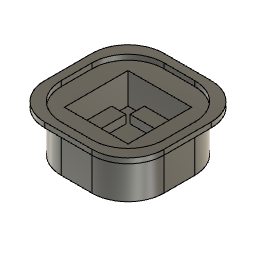
buttonCap (Autodesk Fusion 360 design; units mm, degrees)
Autodesk Fusion 360 part; units mm, degrees
sketch "Esquisse1" plane through (0, 0, 0) normal (0, 0, 1) x (1, 0, 0)
  line L0 (3.5, 0) -> (6.5, 0)
  line L1 (10, -3.5) -> (10, -6.5)
  line L2 (6.5, -10) -> (3.5, -10)
  line L3 (0, -6.5) -> (0, -3.5)
  arc A0 (3.5, 0) -> (0, -3.5) centre (3.5, -3.5) ccw
  arc A1 (10, -3.5) -> (6.5, 0) centre (6.5, -3.5) ccw
  arc A2 (6.5, -10) -> (10, -6.5) centre (6.5, -6.5) ccw
  arc A3 (0, -6.5) -> (3.5, -10) centre (3.5, -6.5) ccw
  point P0 (10, 0)
  point P1 (0, -10)
  dimension "d2" = 10
  dimension "d3" = 10
  dimension "d4" = 3.5
  dimension "d6" = 3.5
  dimension "d7" = 3.5
  dimension "d8" = 3.5
  constraint horizontal L0
  constraint vertical L1
  constraint horizontal L2
  constraint vertical L3
  constraint coincident origin L0
  constraint coincident origin L3
  constraint tangent L0 A0
  constraint tangent L3 A0
  constraint coincident P0 L0
  constraint coincident P0 L1
  constraint tangent L0 A1
  constraint tangent L1 A1
  constraint tangent L1 A2
  constraint tangent L2 A2
  constraint coincident P1 L2
  constraint coincident P1 L3
  constraint tangent L2 A3
  constraint tangent L3 A3
  measures "d2" distance of origin P0
  measures "d3" distance of origin P1
  measures "d4" radius of A0
  measures "d6" radius of A1
  measures "d7" radius of A2
  measures "d8" radius of A3
extrude "Extrusion1" add sketch "Esquisse1" along normal blind 4
ref_plane "Plan de construction1" through (0, 0, 4) normal (0, 0, 1) x (1, 0, 0)
sketch "button" plane through (0, 0, 4) normal (0, 0, 1) x (1, 0, 0)
  line L0 (0, 0) -> (1.9, 0) construction
  line L1 (0, 0) -> (0, -1.9) construction
  line L2 (1.9, 0) -> (1.9, -10) construction
  line L3 (0, -1.9) -> (10, -1.9) construction
  line L4 (1.9, -1.9) -> (8.1, -1.9)
  line L5 (8.1, -1.9) -> (8.1, -8.1)
  line L6 (8.1, -8.1) -> (1.9, -8.1)
  line L7 (1.9, -8.1) -> (1.9, -1.9)
  point P0 (1.9, -1.9)
  dimension "d14" = 1.9
  dimension "d15" = 1.9
  dimension "d16" = 10
  dimension "d17" = 10
  dimension "d18" = 6.2
  dimension "d19" = 6.2
  constraint coincident L0.start L1.start
  constraint horizontal L0
  constraint perpendicular L0 L1
  constraint perpendicular L0 L2
  constraint perpendicular L1 L3
  constraint coincident L2 P0
  constraint coincident L3 P0
  constraint horizontal L4
  constraint vertical L5
  constraint horizontal L6
  constraint vertical L7
  constraint coincident P0 L4.start
  measures "d14" distance of L0.start L0.end
  measures "d15" distance of L0.start L1.end
  measures "d16" distance of L0.end L2.end
  measures "d17" distance of L1.end L3.end
  measures "d18" distance of P0 L4.end
  measures "d19" distance of P0 L6.end
extrude "Extrude2" cut sketch "button" against normal blind 3
ref_plane "WorkPlane2" through (0, 0, 1) normal (0, 0, 1) x (1, 0, 0)
sketch "buttonHolder" plane through (0, 0, 1) normal (0, 0, 1) x (1, 0, 0)
  line L0 (0, 0) -> (3.5, 0) construction
  line L1 (0, 0) -> (0, -1.9) construction
  line L2 (3.5, 0) -> (3.5, -10) construction
  line L3 (0, -1.9) -> (10, -1.9) construction
  line L4 (3.5, -1.9) -> (6.5, -1.9)
  line L5 (6.5, -1.9) -> (6.5, -3.3)
  line L6 (6.5, -3.3) -> (3.5, -3.3)
  line L7 (3.5, -3.3) -> (3.5, -1.9)
  line L8 (0, 0) -> (0, -8.1) construction
  line L9 (0, -8.1) -> (10, -8.1) construction
  line L10 (3.5, -8.1) -> (6.5, -8.1)
  line L11 (6.5, -8.1) -> (6.5, -6.7)
  line L12 (6.5, -6.7) -> (3.5, -6.7)
  line L13 (3.5, -6.7) -> (3.5, -8.1)
  line L14 (0, 0) -> (1.9, 0) construction
  line L15 (1.9, 0) -> (1.9, -3.5) construction
  line L16 (1.9, -3.5) -> (3.3, -3.5)
  line L17 (3.3, -3.5) -> (3.3, -6.5)
  line L18 (3.3, -6.5) -> (1.9, -6.5)
  line L19 (1.9, -6.5) -> (1.9, -3.5)
  line L20 (0, 0) -> (8.1, 0) construction
  line L21 (8.1, 0) -> (8.1, -3.5) construction
  line L22 (8.1, -3.5) -> (6.7, -3.5)
  line L23 (6.7, -3.5) -> (6.7, -6.5)
  line L24 (6.7, -6.5) -> (8.1, -6.5)
  line L25 (8.1, -6.5) -> (8.1, -3.5)
  point P0 (3.5, -1.9)
  point P1 (3.5, -8.1)
  dimension "d25" = 3.5
  dimension "d26" = 1.9
  dimension "d27" = 10
  dimension "d28" = 10
  dimension "d29" = 3
  dimension "d30" = 1.4
  dimension "d32" = 8.1
  dimension "d33" = 10
  dimension "d34" = 3
  dimension "d35" = 1.4
  dimension "d36" = 1.9
  dimension "d37" = 3.5
  dimension "d38" = 1.4
  dimension "d39" = 3
  dimension "d40" = 8.1
  dimension "d41" = 3.5
  dimension "d42" = 1.4
  dimension "d43" = 3
  constraint coincident L0.start L1.start
  constraint horizontal L0
  constraint perpendicular L0 L1
  constraint perpendicular L0 L2
  constraint perpendicular L1 L3
  constraint coincident L2 P0
  constraint coincident L3 P0
  constraint horizontal L4
  constraint vertical L5
  constraint horizontal L6
  constraint vertical L7
  constraint coincident P0 L4.start
  constraint perpendicular L3 L8
  constraint perpendicular L2 L9
  constraint coincident L2 P1
  constraint coincident L9 P1
  constraint horizontal L10
  constraint vertical L11
  constraint horizontal L12
  constraint vertical L13
  constraint coincident P1 L10.start
  constraint perpendicular L8 L14
  constraint perpendicular L0 L15
  constraint horizontal L16
  constraint vertical L17
  constraint horizontal L18
  constraint vertical L19
  constraint perpendicular L8 L20
  constraint perpendicular L20 L21
  constraint horizontal L22
  constraint vertical L23
  constraint horizontal L24
  constraint vertical L25
  measures "d25" distance of L0.start L0.end
  measures "d26" distance of L0.start L1.end
  measures "d27" distance of L0.end L2.end
  measures "d28" distance of L1.end L3.end
  measures "d29" distance of P0 L4.end
  measures "d30" distance of P0 L6.end
  measures "d32" distance of L0.start L8.end
  measures "d33" distance of L8.end L9.end
  measures "d34" distance of P1 L10.end
  measures "d35" distance of P1 L12.end
  measures "d36" distance of L0.start L14.end
  measures "d37" distance of L14.end L15.end
  measures "d38" distance of L15.end L16.end
  measures "d39" distance of L15.end L18.end
  measures "d40" distance of L0.start L20.end
  measures "d41" distance of L20.end L21.end
  measures "d42" distance of L21.end L22.end
  measures "d43" distance of L21.end L24.end
extrude "Extrude3" add sketch "buttonHolder" along normal blind 0.8
sketch "collar" plane through (0, 0, 4) normal (0, 0, 1) x (1, 0, 0)
  line L0 (2.7, 0.8) -> (7.3, 0.8)
  line L1 (-0.8, -7.3) -> (-0.8, -2.7)
  line L2 (10.8, -2.7) -> (10.8, -7.3)
  arc A0 (10.8, -2.7) -> (7.3, 0.8) centre (7.3, -2.7) ccw
  line L3 (7.3, -10.8) -> (2.7, -10.8)
  arc A1 (7.3, -10.8) -> (10.8, -7.3) centre (7.3, -7.3) ccw
  arc A2 (2.7, 0.8) -> (-0.8, -2.7) centre (2.7, -2.7) ccw
  arc A3 (-0.8, -7.3) -> (2.7, -10.8) centre (2.7, -7.3) ccw
  line L4 (0, 0) -> (-0.8, 0) construction
  line L5 (-0.8, 0) -> (-0.8, 0.8) construction
  line L6 (-0.8, 0.8) -> (0, 0.8) construction
  line L7 (0, 0.8) -> (0, 0) construction
  point P0 (10.8, 0.8)
  point P1 (-0.8, -10.8)
  point P2 (-0.8, 0.8)
  point P3 (-0.8, 0.8)
  dimension "d47" = 11.6
  dimension "d48" = 11.6
  dimension "d49" = 3.5
  dimension "d50" = 3.5
  dimension "d51" = 3.5
  dimension "d52" = 3.5
  dimension "d54" = 0.8
  dimension "d55" = 0.8
  constraint horizontal L0
  constraint vertical L2
  constraint horizontal L3
  constraint vertical L1
  constraint coincident P3 P2
  constraint coincident P3 L0
  constraint coincident P3 L1
  constraint tangent L0 A2
  constraint tangent L1 A2
  constraint coincident P0 L0
  constraint coincident P0 L2
  constraint tangent L0 A0
  constraint tangent L2 A0
  constraint tangent L2 A1
  constraint tangent L3 A1
  constraint coincident P1 L3
  constraint coincident P1 L1
  constraint tangent L3 A3
  constraint tangent L1 A3
  constraint horizontal L4
  constraint vertical L5
  constraint horizontal L6
  constraint vertical L7
  constraint coincident L4.start L7.end
  measures "d47" distance of P0 P3
  measures "d48" distance of P1 P3
  measures "d49" radius of A2
  measures "d50" radius of A0
  measures "d51" radius of A1
  measures "d52" radius of A3
  measures "d54" distance of L4.start L4.end
  measures "d55" distance of L4.start L6.end
extrude "Extrude4" add sketch "collar" along normal blind 0.5
sketch "innerCollar" plane through (0, 0, 4) normal (0, 0, 1) x (1, 0, 0)
  line L0 (6.5, -10) -> (3.5, -10)
  arc A0 (0, -6.5) -> (3.5, -10) centre (3.5, -6.5) ccw
  arc A1 (6.5, -10) -> (10, -6.5) centre (6.5, -6.5) ccw
  arc A2 (3.5, 0) -> (0, -3.5) centre (3.5, -3.5) ccw
  line L1 (10, -3.5) -> (10, -6.5)
  arc A3 (10, -3.5) -> (6.5, 0) centre (6.5, -3.5) ccw
  line L2 (0, -6.5) -> (0, -3.5)
  line L3 (3.5, 0) -> (6.5, 0)
  point P0 (10, 0)
  point P1 (0, -10)
  dimension "d59" = 10
  dimension "d60" = 10
  dimension "d61" = 3.5
  dimension "d62" = 3.5
  dimension "d63" = 3.5
  dimension "d64" = 3.5
  constraint horizontal L3
  constraint vertical L1
  constraint horizontal L0
  constraint vertical L2
  constraint coincident origin L3
  constraint coincident origin L2
  constraint tangent A2 L3
  constraint tangent A2 L2
  constraint coincident P0 L3
  constraint coincident P0 L1
  constraint tangent A3 L3
  constraint tangent L1 A3
  constraint tangent A1 L1
  constraint tangent L0 A1
  constraint coincident P1 L0
  constraint coincident P1 L2
  constraint tangent L0 A0
  constraint tangent A0 L2
  measures "d59" distance of P0 origin
  measures "d60" distance of P1 origin
  measures "d61" radius of A2
  measures "d62" radius of A3
  measures "d63" radius of A1
  measures "d64" radius of A0
extrude "Extrude5" cut sketch "innerCollar" along normal blind 0.5
equation "capSize = 10 mm"
equation "d2 = capSize"
equation "d3 = capSize"
equation "d4 = capRadius"
equation "capRadius = 3.5 mm"
equation "d6 = capRadius"
equation "d7 = capRadius"
equation "d8 = capRadius"
equation "d9 = capHeight"
equation "capHeight = 4 mm"
equation "d12 = capHeight"
equation "buttonSize = 6.2 mm"
equation "d14 = ( capSize - buttonSize ) / 2"
equation "d15 = ( capSize - buttonSize ) / 2"
equation "d16 = capSize"
equation "d17 = capSize"
equation "d18 = buttonSize"
equation "d19 = buttonSize"
equation "d20 = -buttonHeight"
equation "buttonHeight = 3 mm"
equation "d23 = -buttonHeight"
equation "buttonHolderLength = 3 mm"
equation "d25 = ( capSize - buttonHolderLength ) / 2"
equation "d26 = ( capSize - buttonSize ) / 2"
equation "d27 = capSize"
equation "d28 = capSize"
equation "d29 = buttonHolderLength"
equation "d30 = buttonHolderWidth"
equation "buttonHolderWidth = 1.4 mm"
equation "d32 = capSize - ( ( capSize - buttonSize ) / 2 )"
equation "d33 = capSize"
equation "d34 = buttonHolderLength"
equation "d35 = buttonHolderWidth"
equation "d36 = ( capSize - buttonSize ) / 2"
equation "d37 = ( capSize - buttonHolderLength ) / 2"
equation "d38 = buttonHolderWidth"
equation "d39 = buttonHolderLength"
equation "d40 = capSize - ( ( capSize - buttonSize ) / 2 )"
equation "d41 = ( capSize - buttonHolderLength ) / 2"
equation "d42 = buttonHolderWidth"
equation "d43 = buttonHolderLength"
equation "buttonHolderHeight = 0.8 mm"
equation "d45 = buttonHolderHeight"
equation "d47 = capSize + ( 2 * collarSize )"
equation "d48 = capSize + ( 2 * collarSize )"
equation "d49 = capRadius"
equation "d50 = capRadius"
equation "d51 = capRadius"
equation "d52 = capRadius"
equation "collarSize = 0.8 mm"
equation "d54 = collarSize"
equation "d55 = collarSize"
equation "collarHeight = 0.5 mm"
equation "d57 = collarHeight"
equation "d59 = capSize"
equation "d60 = capSize"
equation "d61 = capRadius"
equation "d62 = capRadius"
equation "d63 = capRadius"
equation "d64 = capRadius"
equation "d65 = collarHeight"
